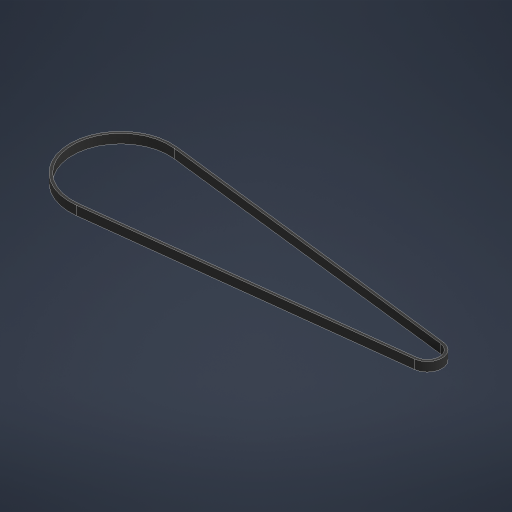
# Autodesk Inventor part: CORL_017_BodyBelt
Saved by Autodesk Inventor 2024.2 (Build 282272000, 272)
## iProperties
Created: 2024-08-06
Part Number: CORL_017_BodyBelt
Material: Rubber, Silicone
Document SubType Name: Modeling
Designer: Bryan
Density: 1.25 g/cm^3
Appearance: Rubber - Black
Author: Bryan
Autodesk Inventor part; units mm, degrees
ref_plane "YZ Plane" through (0, 0, 0) normal (1, 0, 0) x (0, 1, 0)
ref_plane "XZ Plane" through (0, 0, 0) normal (0, 1, 0) x (-1, 0, 0)
ref_plane "XY Plane" through (0, 0, 0) normal (0, 0, 1) x (1, 0, 0)
sketch "Sketch1" plane through (0, 0, 0) normal (0, 1, 0) x (-1, 0, 0)
  circle A0 centre (304.1396, 0) radius 47.752 construction
  line L0 (298.5166, 47.4198) -> (-1.4058, 11.8549)
  line L1 (298.5166, -47.4198) -> (-1.4058, -11.8549)
  arc A1 (298.5166, -47.4198) -> (298.5166, 47.4198) centre (304.1396, 0) ccw
  arc A2 (-1.4058, 11.8549) -> (-1.4058, -11.8549) centre (0, 0) ccw
  line L2 (-1.7049, 14.3773) -> (298.2175, 49.9421)
  arc A3 (298.2175, -49.9421) -> (298.2175, 49.9421) centre (304.1396, 0) ccw
  line L3 (298.2175, -49.9421) -> (-1.7049, -14.3773)
  arc A4 (-1.7049, 14.3773) -> (-1.7049, -14.3773) centre (0, 0) ccw
  dimension "d1" = 95.504
  dimension "d2" = 304.1396
  dimension "d3" = 11.938
  dimension "d4" = 2.54
  constraints: 10 point on circle, 8 end point, 6 tangent, 5 centre point, 1 coincident, 1 horizontal alignment, 3 other
  measures "d1" diameter of A0
  measures "d2" distance of point (0, 0) A0.centre
  measures "d3" radius of A2
  measures "d4" distance between parallel lines of L0 L2
extrude "Extrusion1" add sketch "Sketch1" along normal blind 9
body "Solid1"
